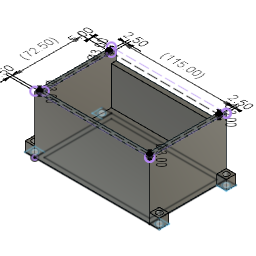
Board_Bottom v7 (Autodesk Fusion 360 design; units mm, degrees)
Autodesk Fusion 360 part; units mm, degrees
sketch "Sketch1" plane through (0, 0, 0) normal (0, 0, 1) x (1, 0, 0)
  line L0 (0, 0) -> (120, 0)
  line L1 (120, 0) -> (120, 80)
  line L2 (120, 80) -> (0, 80)
  line L3 (0, 80) -> (0, 0)
  line L4 (120, 80) -> (130, 80)
  line L5 (130, 80) -> (130, 70)
  line L6 (130, 70) -> (120, 70)
  line L7 (120, 70) -> (120, 80)
  line L8 (120, 0) -> (130, 0)
  line L9 (130, 0) -> (130, 10)
  line L10 (130, 10) -> (120, 10)
  line L11 (120, 10) -> (120, 0)
  line L12 (0, 0) -> (-10, 0)
  line L13 (-10, 0) -> (-10, 10)
  line L14 (-10, 10) -> (0, 10)
  line L15 (0, 10) -> (0, 0)
  line L16 (0, 80) -> (-10, 80)
  line L17 (-10, 80) -> (-10, 70)
  line L18 (-10, 70) -> (0, 70)
  line L19 (0, 70) -> (0, 80)
  circle A0 centre (125, 75) radius 3
  circle A1 centre (125, 5) radius 3
  circle A2 centre (-5, 75) radius 3
  circle A3 centre (-5, 5) radius 3
  line L20 (115, 75) -> (5, 75)
  line L21 (5, 75) -> (5, 5)
  line L22 (5, 5) -> (115, 5)
  line L23 (115, 5) -> (115, 75)
  dimension "d1" = 80
  dimension "d2" = 120
  dimension "d3" = 6
  dimension "d4" = 6
  dimension "d5" = 6
  dimension "d6" = 6
  dimension "d7" = -5
  constraint horizontal L0
  constraint vertical L1
  constraint horizontal L2
  constraint vertical L3
  constraint coincident L0.start L3.end
  constraint horizontal L4
  constraint vertical L5
  constraint horizontal L6
  constraint vertical L7
  constraint horizontal L8
  constraint vertical L9
  constraint horizontal L10
  constraint vertical L11
  constraint horizontal L12
  constraint vertical L13
  constraint horizontal L14
  constraint vertical L15
  constraint horizontal L16
  constraint vertical L17
  constraint horizontal L18
  constraint vertical L19
  measures "d1" distance of L0.start L2.end
  measures "d2" distance of L1.end L2.end
  measures "d3" diameter of A0
  measures "d4" diameter of A1
  measures "d5" diameter of A2
  measures "d6" diameter of A3
extrude "Extrude2" add sketch "Sketch1" along normal blind 60 contours L0 L1 L2 L3 L7 L11 L15 L19 makes body 1
extrude "Extrude1" add sketch "Sketch1" along normal blind 10 separate body contours L3 L12 L13 L14 L15 | L1 L8 L9 L10 L11 | L3 L16 L17 L18 L19 | L1 L4 L5 L6 L7 | L20 L21 L22 L23 makes body 2 at (123.6314, 2.3304, 3.3333) makes body 3 at (127.6347, 76.4348, 3.3333) makes body 4 at (-2.0037, 4.8505, 6.6667) makes body 5 at (-2.1809, 73.9739, 6.6667) makes body 6 at (41.6667, 28.3333, 0)
sketch "Sketch2" plane through (0, 80, 0) normal (0, 1, 0) x (-1, 0, 0)
  line L0 (-120, 0) -> (0, 0)
  line L1 (0, 0) -> (0, 60)
  line L2 (0, 60) -> (-120, 60)
  line L3 (-120, 60) -> (-120, 0)
  line L4 (-115.0684, 60) -> (-5, 60)
  line L5 (-5, 60) -> (-5, 50)
  line L6 (-5, 50) -> (-115.0684, 50)
  line L7 (-115.0684, 50) -> (-115.0684, 60)
  constraint horizontal L4
  constraint vertical L5
  constraint horizontal L6
  constraint vertical L7
  constraint coincident L2 L4.start
extrude "Extrude3" cut sketch "Sketch2" against normal up to surface (5 mm away) contours L2 L4 L5 L6 L7 bodies 1
sketch "Sketch3" plane through (0, 80, 0) normal (0, 1, 0) x (-1, 0, 0)
  line L0 (-115.0684, 50) -> (-115.0684, 60)
  line L1 (-115.0684, 60) -> (-120, 60)
  line L2 (-120, 60) -> (-120, 0)
  line L3 (-120, 0) -> (0, 0)
  line L4 (0, 0) -> (0, 60)
  line L5 (0, 60) -> (-5, 60)
  line L6 (-5, 60) -> (-5, 50)
  line L7 (-5, 50) -> (-115.0684, 50)
sketch "Sketch4" plane through (0, 0, 60) normal (0, 0, 1) x (-1, 0, 0)
  line L0 (-115.0684, -80) -> (-115.0684, -75)
  line L1 (-115.0684, -75) -> (-115, -75)
  line L2 (-115, -75) -> (-115, -5)
  line L3 (-115, -5) -> (-5, -5)
  line L4 (-5, -5) -> (-5, -80)
  line L5 (-5, -80) -> (0, -80)
  line L6 (0, -80) -> (0, 0)
  line L7 (0, 0) -> (-120, 0)
  line L8 (-120, 0) -> (-120, -80)
  line L9 (-120, -80) -> (-115.0684, -80)
  line L10 (-2.5, -75) -> (-117.5, -75) construction
  line L11 (-117.5, -75) -> (-117.5, -2.5) construction
  line L12 (-117.5, -2.5) -> (-2.5, -2.5) construction
  line L13 (-2.5, -2.5) -> (-2.5, -75) construction
  line L14 (-5, -75) -> (-5, -5) construction
  line L15 (0, 0) -> (-120, 0) construction
  line L16 (-120, 0) -> (-120, -80) construction
  line L17 (-120, -80) -> (0, -80) construction
  circle A0 centre (-2.5, -75) radius 1.5
  circle A1 centre (-2.5, -2.5) radius 1.5
  circle A2 centre (-117.5, -2.5) radius 1.5
  circle A3 centre (-117.5, -75) radius 1.5
  dimension "d15" = 2.5
  dimension "d16" = 2.5
  dimension "d17" = 2.5
  dimension "d18" = 5
  dimension "d19" = 115
  dimension "d20" = 72.5
  dimension "d22" = 3
  dimension "d23" = 3
  dimension "d24" = 3
  dimension "d25" = 3
  constraint horizontal L10
  constraint vertical L11
  constraint horizontal L12
  constraint vertical L13
  constraint coincident L10.start L13.end
  constraint coincident L12.end L13.start
  constraint coincident L11.end L12.start
  constraint coincident L10.end L11.start
  measures "d15" distance of L13 L14
  measures "d16" distance of L12 L15
  measures "d17" distance of L11 L16
  measures "d18" distance of L10 L17
  measures "d19" distance of L10.start L10.end
  measures "d20" distance of L10.start L12.end
  measures "d22" diameter of A0
  measures "d23" diameter of A1
  measures "d24" diameter of A2
  measures "d25" diameter of A3
extrude "Extrude4" [suppressed]
sketch "Sketch5" plane through (0, 0, 10) normal (0, 0, 1) x (-1, 0, 0)
  line L0 (-115, -5) -> (-115, -75)
  line L1 (-115, -75) -> (-5, -75)
  line L2 (-5, -75) -> (-5, -5)
  line L3 (-5, -5) -> (-115, -5)
  line L4 (-10, -10) -> (-110, -10) construction
  line L5 (-110, -10) -> (-110, -70) construction
  line L6 (-110, -70) -> (-10, -70) construction
  line L7 (-10, -70) -> (-10, -10) construction
  line L8 (-10, -60) -> (-110, -60) construction
  line L9 (-10, -50) -> (-110, -50) construction
  line L10 (-10, -40) -> (-110, -40) construction
  line L11 (-10, -30) -> (-110, -30) construction
  line L12 (-10, -20) -> (-110, -20) construction
  circle A0 centre (-10, -60) radius 1.5
  circle A1 centre (-10, -50) radius 1.5
  circle A2 centre (-10, -40) radius 1.5
  circle A3 centre (-10, -30) radius 1.5
  circle A4 centre (-10, -20) radius 1.5
  dimension "d28" = -5
  dimension "d29" = 10
  dimension "d30" = 3
  dimension "d31" = 3
  dimension "d32" = 3
  dimension "d33" = 3
  dimension "d34" = 3
  constraint coincident L7 L8.start
  constraint coincident L5 L8.end
  constraint perpendicular L5 L8
  constraint coincident L7 L9.start
  constraint coincident L5 L9.end
  constraint perpendicular L5 L9
  constraint midpoint L7 L10.start
  constraint midpoint L5 L10.end
  constraint coincident L7 L11.start
  constraint coincident L5 L11.end
  constraint perpendicular L5 L11
  constraint coincident L7 L12.start
  constraint coincident L5 L12.end
  constraint perpendicular L7 L12
  constraint coincident L8.start A0.centre
  constraint coincident L9.start A1.centre
  constraint coincident L10.start A2.centre
  constraint coincident L11.start A3.centre
  constraint coincident L12.start A4.centre
  measures "d29" distance of L6 L8
  measures "d30" diameter of A0
  measures "d31" diameter of A1
  measures "d32" diameter of A2
  measures "d33" diameter of A3
  measures "d34" diameter of A4
extrude "Extrude5" [suppressed]
pattern_linear "R-Pattern1" [suppressed]
sketch "Sketch6" plane through (120, 0, 0) normal (1, 0, 0) x (0, 1, 0)
  line L0 (0, 0) -> (80, 0)
  line L1 (80, 0) -> (80, 60)
  line L2 (80, 60) -> (0, 60)
  line L3 (0, 60) -> (0, 0)
  circle A0 centre (40, 25) radius 10
  dimension "d41" = 20
  measures "d41" diameter of A0
extrude "Extrude6" [suppressed]
fillet "Fillet1" [suppressed]
fillet "Fillet2" [suppressed]
